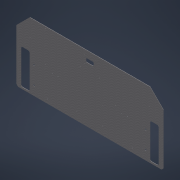
# Autodesk Inventor part: PlanchaBaseInferior
Saved by Autodesk Inventor 2022 (Build 260153000, 153)
## iProperties
Created: 2021-09-22
Part Number: PlanchaBaseInferior
Material: Steel, Mild, Welded
Document SubType Name: Sheet Metal
Designer: Andres
Density: 7.85 g/cm^3
Sheet Metal Rule: Default_mm
Appearance: Weld - Steel Mild
Author: Andres
Autodesk Inventor part; units mm, degrees
ref_plane "YZ Plane" through (0, 0, 0) normal (1, 0, 0) x (0, 1, 0)
ref_plane "XZ Plane" through (0, 0, 0) normal (0, 1, 0) x (-1, 0, 0)
ref_plane "XY Plane" through (0, 0, 0) normal (0, 0, 1) x (1, 0, 0)
sketch "Sketch1" plane through (0, 0, 0) normal (0, 0, 1) x (1, 0, 0)
  line L0 (725.9853, -345.9853) -> (570.9853, -345.9853) construction
  line L1 (725.9853, -370.9853) -> (570.9853, -370.9853) construction
  line L2 (125.9853, -345.9853) -> (750.9853, -345.9853)
  line L3 (750.9853, -345.9853) -> (933.3076, -345.9853)
  line L4 (933.3076, -345.9853) -> (945.9853, -333.3076)
  line L5 (945.9853, -333.3076) -> (945.9853, 16.337)
  line L6 (945.9853, 16.337) -> (853.3076, 109.0147)
  line L7 (853.3076, 109.0147) -> (23.663, 109.0147)
  line L8 (-69.0147, 16.337) -> (23.663, 109.0147)
  line L9 (-69.0147, 16.337) -> (-69.0147, -333.3076)
  line L10 (-69.0147, -333.3076) -> (-56.337, -345.9853)
  line L11 (125.9853, -345.9853) -> (-56.337, -345.9853)
  line L12 (725.9853, -370.9853) -> (725.9853, -345.9853) projected
  line L13 (570.9853, -345.9853) -> (570.9853, -370.9853) projected
  constraints: 20 end point, 2 perpendicular, 1 collinear
extrude "Plate1" add sketch "Sketch1" along normal blind 3
sketch "Sketch2" plane through (0, 0, 3) normal (0, 0, 1) x (1, 0, 0)
  line L0 (-31.5147, -334.9853) -> (-31.5147, -114.9853) projected
  line L1 (18.4853, -114.9853) -> (18.4853, -334.9853) projected
  line L2 (858.4853, -334.9853) -> (858.4853, -114.9853) projected
  line L3 (908.4853, -114.9853) -> (908.4853, -334.9853) projected
  line L4 (-26.5147, -98.1151) -> (13.4853, -98.1151)
  arc A0 (-26.5147, -98.1151) -> (-31.5147, -114.9853) centre (-26.5147, -103.1151) ccw
  arc A1 (18.4853, -114.9853) -> (13.4853, -98.1151) centre (13.4853, -103.1151) ccw
  line L5 (-26.5147, -328.1151) -> (13.4853, -328.1151)
  arc A2 (13.4853, -328.1151) -> (18.4853, -334.9853) centre (13.4853, -323.1151) ccw
  arc A3 (-31.5147, -334.9853) -> (-26.5147, -328.1151) centre (-26.5147, -323.1151) ccw
  arc A4 (903.0889, -328.1151) -> (908.4853, -334.9853) centre (903.0889, -323.1151) ccw
  line L6 (903.0889, -328.1151) -> (863.0889, -328.1151)
  arc A5 (858.4853, -334.9853) -> (863.0889, -328.1151) centre (863.0889, -323.1151) ccw
  arc A6 (908.4853, -114.9853) -> (903.0889, -98.1151) centre (903.0889, -103.1151) ccw
  arc A7 (863.0889, -98.1151) -> (858.4853, -114.9853) centre (863.0889, -103.1151) ccw
  line L7 (903.0889, -98.1151) -> (863.0889, -98.1151)
  line L8 (23.4853, -323.1151) -> (23.4853, -103.1151)
  arc A8 (23.4853, -103.1151) -> (13.4853, -93.1151) centre (13.4853, -103.1151) ccw
  line L9 (13.4853, -93.1151) -> (-26.5147, -93.1151)
  arc A9 (-26.5147, -93.1151) -> (-36.5147, -103.1151) centre (-26.5147, -103.1151) ccw
  line L10 (-36.5147, -103.1151) -> (-36.5147, -323.1151)
  arc A10 (-36.5147, -323.1151) -> (-26.5147, -333.1151) centre (-26.5147, -323.1151) ccw
  line L11 (-26.5147, -333.1151) -> (13.4853, -333.1151)
  arc A11 (13.4853, -333.1151) -> (23.4853, -323.1151) centre (13.4853, -323.1151) ccw
  line L12 (913.0889, -323.1151) -> (913.0889, -103.1151)
  arc A12 (913.0889, -103.1151) -> (903.0889, -93.1151) centre (903.0889, -103.1151) ccw
  line L13 (903.0889, -93.1151) -> (863.0889, -93.1151)
  arc A13 (863.0889, -93.1151) -> (853.0889, -103.1151) centre (863.0889, -103.1151) ccw
  line L14 (853.0889, -103.1151) -> (853.0889, -323.1151)
  arc A14 (853.0889, -323.1151) -> (863.0889, -333.1151) centre (863.0889, -323.1151) ccw
  line L15 (863.0889, -333.1151) -> (903.0889, -333.1151)
  arc A15 (903.0889, -333.1151) -> (913.0889, -323.1151) centre (903.0889, -323.1151) ccw
  line L16 (33.4853, -313.1151) -> (73.4853, -313.1151)
  line L17 (33.4853, -143.1151) -> (73.4853, -143.1151)
  line L18 (843.4853, -143.1151) -> (803.4853, -143.1151)
  line L19 (803.4853, -313.1151) -> (843.4853, -313.1151)
  line L20 (33.4853, 101.5147) -> (33.4853, -338.4853) projected
  line L21 (73.4853, 101.5147) -> (73.4853, -338.4853) projected
  line L22 (803.4853, -338.4853) -> (803.4853, 101.5147) projected
  line L23 (843.4853, -338.4853) -> (843.4853, 101.5147) projected
  point P0 (438.4853, 79.5147)
  dimension "d19" = 5
  dimension "d20" = 5
  dimension "d21" = 20
  dimension "d22" = 50
  dimension "d23" = 50
  dimension "d24" = 20
  constraints: 32 end point, 16 point on circle, 8 centre point, 8 point on line, 5 horizontal, 62 other
  measures "d19" distance between parallel lines of L1 L8
  measures "d21" distance between parallel lines of L11 L16
  measures "d22" distance between parallel lines of L9 L17
  measures "d23" distance between parallel lines of L13 L18
  measures "d24" distance between parallel lines of L19 L15
extrude "Cut1" cut sketch "Sketch2" against normal through all contours A10 L10 A9 L9 A8 A1 L4 A0 L0 | L0 A0 L4 A1 A8 L8 L1 A2 L5 A3 L11 A10 | A3 L5 A2 L1 A11 L11 | L1 A2 A11 | L1 A1 L8 A11 A2 | A14 L14 A13 L13 A12 A6 L7 A7 L2 | L2 A7 L7 A6 A12 L12 L3 A4 L6 A5 L15 A14 | A5 L6 A4 L3 A15 L15 | L3 A4 A15 | L3 A6 L12 A15 A4 picked at (18.5475, -330.9544) picked at (908.5177, -331.0591)
sketch "Sketch4" plane through (0, 0, 3) normal (0, 0, 1) x (1, 0, 0)
  line L0 (933.3076, -345.9853) -> (-56.337, -345.9853) projected
  line L1 (-56.337, -345.9853) -> (933.3076, -345.9853) construction
  line L2 (438.4853, 109.0147) -> (438.4853, 49.0147) construction
  line L3 (401.4853, 21.0147) -> (475.4853, 21.0147) construction
  line L4 (475.4853, 21.0147) -> (475.4853, 77.0147) construction
  line L5 (475.4853, 77.0147) -> (401.4853, 77.0147) construction
  line L6 (401.4853, 77.0147) -> (401.4853, 21.0147) construction
  line L7 (401.4853, 21.0147) -> (475.4853, 77.0147) construction
  line L8 (475.4853, 21.0147) -> (401.4853, 77.0147) construction
  line L9 (411.4853, 36.5147) -> (465.4853, 36.5147)
  line L10 (465.4853, 36.5147) -> (465.4853, 61.5147)
  line L11 (465.4853, 61.5147) -> (411.4853, 61.5147)
  line L12 (411.4853, 61.5147) -> (411.4853, 36.5147)
  line L13 (411.4853, 36.5147) -> (465.4853, 61.5147) construction
  line L14 (465.4853, 36.5147) -> (411.4853, 61.5147) construction
  line L15 (23.663, 109.0147) -> (853.3076, 109.0147) projected
  point P0 (0, 0)
  dimension "d46" = 74
  dimension "d47" = 56
  dimension "d55" = 54
  dimension "d56" = 25
  dimension "d59" = 60
  constraints: 26 end point, 5 midpoint, 4 coincident, 4 parallel, 2 horizontal, 2 perpendicular, 1 vertical
  measures "d46" distance of L5.end L4.end
  measures "d47" distance of L4.end L3.end
  measures "d55" distance between parallel lines of L10 L12
  measures "d56" distance between parallel lines of L11 L9
  measures "d59" distance of L2.start L2.end
hole "Hole1" at (401.4853, 77.0147, 3) at (401.4853, 21.0147, 3) at (475.4853, 21.0147, 3) at (475.4853, 77.0147, 3) direction (0, 0, -1) diameter 3.4 end through all clearance for "Countersunk Flat Head Screw ISO 2009/7046" size "M3" standard "ISO"
extrude "Cut3" cut sketch "Sketch4" against normal blind 3
fillet "Corner Round2" radius 6 4 edges at (411.4853, 61.5147, 1.5) (411.4853, 36.5147, 1.5) (465.4853, 61.5147, 1.5) (465.4853, 36.5147, 1.5)
sketch "Sketch5" plane through (0, 0, 3) normal (0, 0, 1) x (1, 0, 0)
  circle A0 centre (219.1853, -146.4853) radius 3.3 projected
  circle A1 centre (179.1853, -146.4853) radius 3.3 projected
  circle A2 centre (147.6853, -314.4853) radius 3.3 projected
  circle A3 centre (349.1853, -162.9853) radius 3 projected
  circle A4 centre (349.1853, -286.9853) radius 2.2 projected
  arc A5 (34.2552, -163.466) -> (33.5853, -165.966) centre (38.5853, -165.966) ccw projected
  line L0 (33.5853, -175.2353) -> (33.5853, -165.966) projected
  line L1 (73.5853, -175.2353) -> (33.5853, -175.2353) projected
  arc A6 (48.0853, -167.9853) -> (59.0853, -167.9853) centre (53.5853, -167.9853) ccw projected
  line L2 (48.0853, -167.9853) -> (48.0853, -160.9853) projected
  arc A7 (59.0853, -160.9853) -> (48.0853, -160.9853) centre (53.5853, -160.9853) ccw projected
  line L3 (59.0853, -160.9853) -> (59.0853, -167.9853) projected
  line L4 (73.5853, -165.966) -> (73.5853, -175.2353) projected
  arc A8 (73.5853, -165.966) -> (72.9154, -163.466) centre (68.5853, -165.966) ccw projected
  line L5 (72.9154, -163.466) -> (67.0087, -153.2353) projected
  arc A9 (67.0087, -153.2353) -> (40.1619, -153.2353) centre (53.5853, -160.9853) ccw projected
  line L6 (40.1619, -153.2353) -> (34.2552, -163.466) projected
  arc A10 (33.5853, -284.0045) -> (34.2552, -286.5045) centre (38.5853, -284.0045) ccw projected
  line L7 (34.2552, -286.5045) -> (40.1619, -296.7353) projected
  arc A11 (40.1619, -296.7353) -> (67.0087, -296.7353) centre (53.5853, -288.9853) ccw projected
  line L8 (67.0087, -296.7353) -> (72.9154, -286.5045) projected
  arc A12 (72.9154, -286.5045) -> (73.5853, -284.0045) centre (68.5853, -284.0045) ccw projected
  line L9 (73.5853, -274.7353) -> (73.5853, -284.0045) projected
  line L10 (73.5853, -274.7353) -> (33.5853, -274.7353) projected
  arc A13 (59.0853, -281.9853) -> (48.0853, -281.9853) centre (53.5853, -281.9853) ccw projected
  line L11 (59.0853, -281.9853) -> (59.0853, -288.9853) projected
  arc A14 (48.0853, -288.9853) -> (59.0853, -288.9853) centre (53.5853, -288.9853) ccw projected
  line L12 (48.0853, -288.9853) -> (48.0853, -281.9853) projected
  line L13 (33.5853, -284.0045) -> (33.5853, -274.7353) projected
  circle A15 centre (527.7853, -162.9853) radius 2.2 projected
  circle A16 centre (527.7853, -286.9853) radius 3 projected
  arc A17 (843.3853, -165.966) -> (842.7154, -163.466) centre (838.3853, -165.966) ccw projected
  line L14 (842.7154, -163.466) -> (836.8087, -153.2353) projected
  arc A18 (836.8087, -153.2353) -> (809.9619, -153.2353) centre (823.3853, -160.9853) ccw projected
  line L15 (809.9619, -153.2353) -> (804.0552, -163.466) projected
  arc A19 (804.0552, -163.466) -> (803.3853, -165.966) centre (808.3853, -165.966) ccw projected
  line L16 (803.3853, -175.2353) -> (803.3853, -165.966) projected
  line L17 (803.3853, -175.2353) -> (843.3853, -175.2353) projected
  arc A20 (817.8853, -167.9853) -> (828.8853, -167.9853) centre (823.3853, -167.9853) ccw projected
  line L18 (817.8853, -167.9853) -> (817.8853, -160.9853) projected
  arc A21 (828.8853, -160.9853) -> (817.8853, -160.9853) centre (823.3853, -160.9853) ccw projected
  line L19 (828.8853, -160.9853) -> (828.8853, -167.9853) projected
  line L20 (843.3853, -165.966) -> (843.3853, -175.2353) projected
  arc A22 (842.7154, -286.5045) -> (843.3853, -284.0045) centre (838.3853, -284.0045) ccw projected
  line L21 (843.3853, -274.7353) -> (843.3853, -284.0045) projected
  line L22 (803.3853, -274.7353) -> (843.3853, -274.7353) projected
  arc A23 (828.8853, -281.9853) -> (817.8853, -281.9853) centre (823.3853, -281.9853) ccw projected
  line L23 (828.8853, -281.9853) -> (828.8853, -288.9853) projected
  arc A24 (817.8853, -288.9853) -> (828.8853, -288.9853) centre (823.3853, -288.9853) ccw projected
  line L24 (817.8853, -288.9853) -> (817.8853, -281.9853) projected
  line L25 (803.3853, -284.0045) -> (803.3853, -274.7353) projected
  arc A25 (803.3853, -284.0045) -> (804.0552, -286.5045) centre (808.3853, -284.0045) ccw projected
  line L26 (804.0552, -286.5045) -> (809.9619, -296.7353) projected
  arc A26 (809.9619, -296.7353) -> (836.8087, -296.7353) centre (823.3853, -288.9853) ccw projected
  line L27 (836.8087, -296.7353) -> (842.7154, -286.5045) projected
  circle A27 centre (697.7853, -146.4853) radius 3.3 projected
  circle A28 centre (657.7853, -146.4853) radius 3.3 projected
  circle A29 centre (733.7853, -314.4853) radius 3.3 projected
  point P0 (0, 0)
sketch "Sketch6" plane through (0, 0, 0) normal (0, 0, -1) x (-1, 0, 0)
  point P0 (-657.7853, -146.4853)
  point P1 (-697.7853, -146.4853)
  point P2 (-219.1853, -146.4853)
  point P3 (-179.1853, -146.4853)
  point P4 (-733.7853, -314.4853)
  point P5 (-147.6853, -314.4853)
hole "Hole2" at (657.7853, -146.4853, 0) at (697.7853, -146.4853, 0) at (219.1853, -146.4853, 0) at (179.1853, -146.4853, 0) at (733.7853, -314.4853, 0) at (147.6853, -314.4853, 0) direction (0, 0, 1) diameter 6.6 end through all
sketch "Sketch7" plane through (0, 0, 0) normal (0, 0, -1) x (-1, 0, 0)
  point P0 (-527.7853, -162.9853)
  point P1 (-527.7853, -286.9853)
  point P2 (-349.1853, -286.9853)
  point P3 (-349.1853, -162.9853)
hole "Hole3" at (527.7853, -162.9853, 0) at (527.7853, -286.9853, 0) at (349.1853, -286.9853, 0) at (349.1853, -162.9853, 0) direction (0, 0, 1) diameter 4.5 end through all
sketch "Sketch9" plane through (0, 0, 3) normal (0, 0, 1) x (1, 0, 0)
  point P0 (53.5853, -160.9853)
  point P1 (53.5853, -281.9853)
  point P2 (823.3853, -160.9853)
  point P3 (823.3853, -281.9853)
hole "Hole5" at (53.5853, -160.9853, 3) at (53.5853, -281.9853, 3) at (823.3853, -160.9853, 3) at (823.3853, -281.9853, 3) direction (0, 0, -1) diameter 11 end through all
sketch "Sketch10" plane through (0, 0, 0) normal (0, 0, -1) x (-1, 0, 0)
  point P0 (-613.8153, 96.5147)
  point P1 (-851.1853, -11.3153)
  point P2 (-505.9853, -11.3153)
  point P3 (-370.9853, -11.3153)
  point P4 (-133.6153, 96.5147)
  point P5 (-133.6153, -119.1453)
  point P6 (-25.7853, -11.3153)
  point P7 (-613.8153, -119.1453)
hole "Hole6" at (613.8153, 96.5147, 0) at (851.1853, -11.3153, 0) at (505.9853, -11.3153, 0) at (370.9853, -11.3153, 0) at (133.6153, 96.5147, 0) at (133.6153, -119.1453, 0) at (25.7853, -11.3153, 0) at (613.8153, -119.1453, 0) direction (0, 0, 1) diameter 4.5 end through all
equation "\"d6\" = Thickness"
equation "\"d53\" = Thickness"
equation "\"d57\" = Thickness"
equation "\"d0\" = Thickness"
equation "\"BendRadius\" = Thickness"
equation "\"BendReliefWidth\" = Thickness"
equation "\"BendReliefDepth\" = 0.5 * Thickness"
equation "\"CornerReliefSize\" = 4 * Thickness"
equation "\"MinimumRemnant\" = 2 * Thickness"
equation "\"TransitionRadius\" = BendRadius"
equation "\"JacobiRadiusSize\" = BendRadius"
equation "\"GapSize\" = Thickness"
equation "\"Thickness\" = 3"
body "Solid1"
